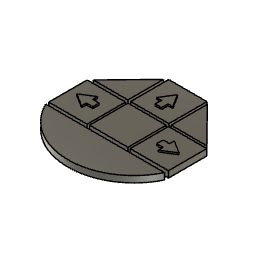
v1 plate model (Autodesk Fusion 360 design; units mm, degrees)
Autodesk Fusion 360 part; units mm, degrees
sketch "Sketch1" plane through (0, 0, 0) normal (0, 0, 1) x (1, 0, 0)
  line L0 (121.8579, 375) -> (-121.8579, 375)
  line L1 (375, 375) -> (-375, -375) construction
  line L2 (-375, 375) -> (375, -375) construction
  line L3 (-132.8792, 117.5215) -> (-372.8792, 117.5215)
  line L4 (-372.8792, 117.5215) -> (-372.8792, -122.4785)
  line L5 (-372.8792, -122.4785) -> (-132.8792, -122.4785)
  line L6 (-132.8792, -122.4785) -> (-132.8792, 117.5215)
  line L7 (-132.8792, 117.5215) -> (-372.8792, -122.4785) construction
  line L8 (-372.8792, 117.5215) -> (-132.8792, -122.4785) construction
  line L9 (120, 120) -> (-120, 120)
  line L10 (-120, 120) -> (-120, -120)
  line L11 (-120, -120) -> (120, -120)
  line L12 (120, -120) -> (120, 120)
  line L13 (120, 120) -> (-120, -120) construction
  line L14 (-120, 120) -> (120, -120) construction
  line L15 (-120.0122, 136.8931) -> (119.9878, 136.8931)
  line L16 (119.9878, 136.8931) -> (119.9878, 376.8931)
  line L17 (119.9878, 376.8931) -> (-120.0122, 376.8931)
  line L18 (-120.0122, 376.8931) -> (-120.0122, 136.8931)
  line L19 (-120.0122, 136.8931) -> (119.9878, 376.8931) construction
  line L20 (119.9878, 136.8931) -> (-120.0122, 376.8931) construction
  line L21 (133.7615, 120) -> (373.7615, 120)
  line L22 (373.7615, 120) -> (373.7615, -120)
  line L23 (373.7615, -120) -> (133.7615, -120)
  line L24 (133.7615, -120) -> (133.7615, 120)
  line L25 (133.7615, 120) -> (373.7615, -120) construction
  line L26 (373.7615, 120) -> (133.7615, -120) construction
  line L27 (135.3754, 135.3754) -> (358.5729, 135.3754)
  line L28 (135.3754, 361.3164) -> (135.3754, 135.3754)
  line L29 (-136.8931, 136.8931) -> (-136.8931, 359.578)
  line L30 (-353.9934, 136.8931) -> (-136.8931, 136.8931)
  line L31 (-371.6745, -142.6376) -> (371.6745, -142.6376)
  arc A0 (-371.6745, -142.6376) -> (371.6745, -142.6376) centre (0, 38.4365) ccw
  line L32 (119.9878, 376.8931) -> (121.8579, 375)
  line L33 (135.3754, 361.3164) -> (358.5729, 135.3754)
  line L34 (-353.9934, 136.8931) -> (-136.8931, 359.578)
  line L35 (-121.8579, 375) -> (-120.0122, 376.8931)
  point P0 (-252.8792, -2.4785)
  point P1 (-252.8792, -2.4785)
  point P2 (-0.0122, 256.8931)
  point P3 (-0.0122, 256.8931)
  point P4 (253.7615, 0)
  point P5 (253.7615, 0)
  dimension "d1" = 750
  dimension "d3" = 750
  dimension "d8" = 240
  dimension "d9" = 240
  dimension "d10" = 240
  dimension "d11" = 240
  dimension "d12" = 240
  dimension "d13" = 240
  dimension "d14" = 240
  dimension "d15" = 240
  constraint horizontal L0
  constraint coincident L1 origin
  constraint coincident L2 origin
  constraint horizontal L3
  constraint perpendicular L3 L4
  constraint parallel L3 L5
  constraint parallel L4 L6
  constraint coincident L7 P1
  constraint coincident L8 P1
  constraint coincident P1 P0
  constraint horizontal L9
  constraint perpendicular L9 L10
  constraint parallel L9 L11
  constraint parallel L10 L12
  constraint coincident L13 origin
  constraint coincident L14 origin
  constraint horizontal L15
  constraint perpendicular L15 L16
  constraint parallel L15 L17
  constraint parallel L16 L18
  constraint coincident L19 P3
  constraint coincident L20 P3
  constraint coincident P3 P2
  constraint horizontal L21
  constraint perpendicular L21 L22
  constraint parallel L21 L23
  constraint parallel L22 L24
  constraint coincident L25 P5
  constraint coincident L26 P5
  constraint coincident P5 P4
  constraint coincident L0.end L34
  constraint coincident L1 L27.start
  constraint parallel L21 L27
  constraint coincident L28.start L32
  constraint perpendicular L27 L28
  constraint coincident L2 L29.start
  constraint parallel L18 L29
  constraint perpendicular L29 L30
  constraint parallel L23 L31
  constraint collinear L32 L33
  constraint collinear L34 L35
  measures "d1" distance of L1.end L2.end
  measures "d3" distance of L2.start L1.end
  measures "d8" distance of L4.end L5.end
  measures "d9" distance of L3.end L4.end
  measures "d10" distance of L10.end L11.end
  measures "d11" distance of L9.end L10.end
  measures "d12" distance of L16.end L17.end P5
  measures "d13" distance of L15.end L16.end P5
  measures "d14" distance of L22.end L23.end
  measures "d15" distance of L21.end L22.end
extrude "Extrude1" add sketch "Sketch1" along normal blind 40 contours L0 L15 L16 L18 | L3 L4 L5 L6 | L9 L10 L11 L12 | L21 L22 L23 L24 | L27 L28 L33 | L29 L30 L34 | L31 A0 makes body 1 at (-209.2599, 211.1214, 0) makes body 2 at (40, -40, 0) makes body 3 at (-40.0122, 216.2621, 0) makes body 4 at (-292.8792, 37.5215, 0) makes body 5 at (213.7615, -40, 0) makes body 6 at (209.7745, 210.689, 0) makes body 7 at (12.9238, -253.4236, 0)
sketch "Sketch2" plane through (0, 0, 40) normal (0, 0, 1) x (-1, 0, 0)
  line L0 (-133.7615, 120) -> (-373.7615, 120)
  line L1 (-373.7615, 120) -> (-373.7615, -120)
  line L2 (-373.7615, -120) -> (-133.7615, -120)
  line L3 (-133.7615, -120) -> (-133.7615, 120)
  line L4 (-200, -20) -> (-200, 20)
  line L5 (20, -190) -> (-20, -190)
  line L6 (200, -20) -> (200, 20)
  line L7 (200, -20) -> (240, -20)
  line L8 (240, -20) -> (240, -50)
  line L9 (240, -50) -> (320, 0)
  line L10 (320, 0) -> (240, 50)
  line L11 (240, 20) -> (240, 50)
  line L12 (240, 20) -> (200, 20)
  line L13 (200, -20) -> (200, 20)
  line L14 (-200, -20) -> (-240, -20)
  line L15 (-240, -20) -> (-240, -50)
  line L16 (-320, 0) -> (-240, -50)
  line L17 (-320, 0) -> (-240, 50)
  line L18 (-240, 20) -> (-240, 50)
  line L19 (-240, 20) -> (-200, 20)
  line L20 (-200, -20) -> (-200, 20)
  line L21 (20, -190) -> (20, -230)
  line L22 (20, -230) -> (50, -230)
  line L23 (0, -310) -> (50, -230)
  line L24 (0, -310) -> (-50, -230)
  line L25 (-20, -230) -> (-20, -190)
  line L26 (20, -190) -> (-20, -190)
  line L27 (-20, -230) -> (-50, -230)
  constraint parallel L3 L4
  constraint perpendicular L1 L5
  constraint perpendicular L5 L6
  constraint perpendicular L6 L7
  constraint perpendicular L6 L12
  constraint perpendicular L4 L14
  constraint perpendicular L4 L19
  constraint perpendicular L5 L21
  constraint perpendicular L5 L25
extrude "Extrude2" add sketch "Sketch2" along normal blind 10 contours L4 L14 L15 L16 L17 L18 L19 L20 | L5 L21 L22 L23 L24 L25 L26 L27 | L6 L7 L8 L9 L10 L11 L12 L13 bodies 3 4 5
equation "d1 = big_base_width"
equation "big_base_width = 75 cm"
equation "d3 = big_base_width"
equation "big_base_depth = 6 cm"
equation "single_block_width = 21 cm"
equation "single_block_length = 21 cm"
equation "single_block_depth = 6 cm"
